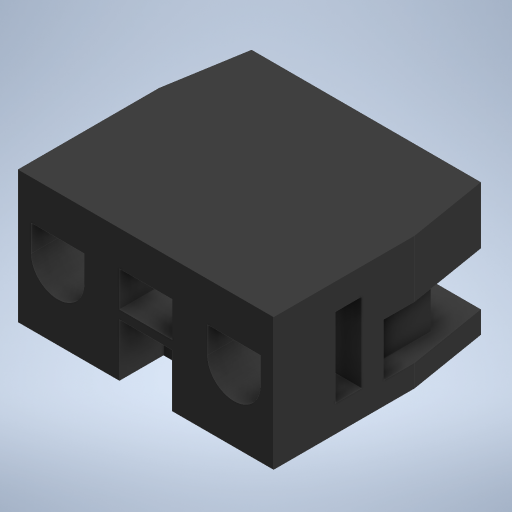
# Autodesk Inventor part: BLOCO DE CONTATO
Saved by Autodesk Inventor 2023 (Build 270158000, 158)
## iProperties
Created: 2023-10-18
Part Number: BLOCO DE CONTATO
Material: Genérico
Document SubType Name: Modeling
Designer: vinicius.sena
Density: 1 g/cm^3
Appearance: Padrão
Author: vinicius.sena
Autodesk Inventor part; units mm, degrees
ref_plane "YZ Plane" through (0, 0, 0) normal (1, 0, 0) x (0, 1, 0)
ref_plane "XZ Plane" through (0, 0, 0) normal (0, 1, 0) x (-1, 0, 0)
ref_plane "XY Plane" through (0, 0, 0) normal (0, 0, 1) x (1, 0, 0)
sketch "Esboço1" plane through (0, 0, 0) normal (0, 0, 1) x (1, 0, 0)
  line L0 (-14.5, 7.5) -> (14.5, 7.5)
  line L1 (14.5, 7.5) -> (14.5, -7.5)
  line L2 (14.5, -7.5) -> (-14.5, -7.5)
  line L3 (-14.5, -7.5) -> (-14.5, 7.5)
  line L4 (-14.5, 7.5) -> (14.5, -7.5) construction
  line L5 (14.5, 7.5) -> (-14.5, -7.5) construction
  point P0 (0, 0)
  dimension "d0" = 29
  dimension "d1" = 15
  constraints: 12 end point, 2 midpoint, 2 parallel, 1 horizontal, 1 perpendicular
  measures "d0" distance of L1.end L2.end
  measures "d1" distance of L0.end L1.end
extrude "Extrusão1" add sketch "Esboço1" along normal blind 25
sketch "Esboço2" plane through (-14.5, 7.5, 0) normal (0, 1, 0) x (1, 0, 0)
  line L0 (0, 0) -> (0, -25) projected
  line L1 (0, 0) -> (0, -9)
  line L2 (29, 0) -> (29, -25) projected
  line L3 (29, 0) -> (29, -9)
  line L4 (1.5, 0) -> (27.5, 0)
  line L5 (27.5, 0) -> (27.5, -9)
  line L6 (27.5, -9) -> (1.5, -9)
  line L7 (1.5, -9) -> (1.5, 0)
  line L8 (1.5, 0) -> (27.5, -9) construction
  line L9 (27.5, 0) -> (1.5, -9) construction
  line L10 (1.5, 0) -> (0, -9)
  line L11 (27.5, 0) -> (29, -9)
  line L12 (29, 0) -> (0, 0) projected
  line L13 (0, 0) -> (0, -25) projected
  line L14 (29, -25) -> (0, -25) projected
  line L15 (29, 0) -> (29, -25) projected
  point P0 (14.5, 0)
  point P1 (14.5, -4.5)
  dimension "d4" = 9
  dimension "d5" = 9
  dimension "d6" = 26
  constraints: 20 end point, 2 midpoint, 2 parallel, 2 point on line, 1 horizontal, 1 perpendicular
  measures "d4" distance of L0.start L1.end
  measures "d5" distance of L2.start L3.end
  measures "d6" distance of L5.end L6.end
extrude "Extrusão2" cut sketch "Esboço2" against normal through all contours L12 L10 L0 | L12 L2 L11
sketch "Esboço3" plane through (0, 0, 25) normal (0, 0, 1) x (1, 0, 0)
  circle A0 centre (10, 0) radius 3
  circle A1 centre (-10, 0) radius 3
  line L0 (-13, -7.5) -> (-13, 7.5) projected
  line L1 (-7, 3) -> (-13, 3)
  line L2 (-13, 3) -> (-13, -3)
  line L3 (-13, -3) -> (-7, -3)
  line L4 (-7, -3) -> (-7, 3)
  line L5 (-7, 3) -> (-13, -3) construction
  line L6 (-13, 3) -> (-7, -3) construction
  line L7 (13, 3) -> (7, 3)
  line L8 (7, 3) -> (7, -3)
  line L9 (7, -3) -> (13, -3)
  line L10 (13, -3) -> (13, 3)
  line L11 (13, 3) -> (7, -3) construction
  line L12 (7, 3) -> (13, -3) construction
  line L13 (3, -1.5) -> (-3, -1.5)
  line L14 (-3, -1.5) -> (-3, -7.5)
  line L15 (-3, -7.5) -> (3, -7.5)
  line L16 (3, -7.5) -> (3, -1.5)
  line L17 (3, -1.5) -> (-3, -7.5) construction
  line L18 (-3, -1.5) -> (3, -7.5) construction
  line L19 (-14.5, -7.5) -> (14.5, -7.5) projected
  point P0 (0, 0)
  point P1 (0, -4.5)
  point P2 (-7, 0)
  point P3 (-13, 0)
  point P4 (7, 0)
  point P5 (13, 0)
  dimension "d9" = 6
  dimension "d10" = 6
  dimension "d11" = 10
  dimension "d12" = 10
  dimension "d13" = 6
  dimension "d14" = 6
  dimension "d15" = 0
  constraints: 36 end point, 6 midpoint, 6 parallel, 3 horizontal, 3 perpendicular, 2 centre point, 2 point on line
  measures "d9" diameter of A0
  measures "d10" diameter of A1
  measures "d11" distance of point (0, 0) A0.centre
  measures "d12" distance of point (0, 0) A1.centre
  measures "d13" distance of L15.end L14.end
  measures "d14" distance of L14.end L13.end
  measures "d15" distance between parallel lines of L19 L15
extrude "Extrusão3" cut sketch "Esboço3" against normal blind 10 contours A0 | A0 L7 L10 | A0 L8 L7 | A1 | A1 L1 L4 | A1 L0 L1
sketch "Esboço4" plane through (-14.5, -7.5, 25) normal (-1, 0, 0) x (0, 0, 1)
  line L0 (-7, 12) -> (-10, 12)
  line L1 (-10, 12) -> (-10, 3)
  line L2 (-10, 3) -> (-7, 3)
  line L3 (-7, 3) -> (-7, 12)
  line L4 (-7, 12) -> (-10, 3) construction
  line L5 (-10, 12) -> (-7, 3) construction
  line L6 (-10, 7.5) -> (-10, 10.5) projected
  point P0 (-25, 7.5)
  point P1 (-8.5, 7.5)
  dimension "d18" = 3
  dimension "d19" = 9
  dimension "d20" = 0
  constraints: 12 end point, 3 midpoint, 2 parallel, 1 horizontal, 1 perpendicular
  measures "d18" distance of L2.end L1.end
  measures "d19" distance of L1.end L0.end
  measures "d20" distance from line of L6 point (-10, 7.5)
extrude "Extrusão4" cut sketch "Esboço4" against normal blind 7.5
sketch "Esboço5" plane through (14.5, -7.5, 25) normal (1, 0, 0) x (0, 0, -1)
  line L0 (7, 3) -> (10, 3)
  line L1 (10, 3) -> (10, 12)
  line L2 (10, 12) -> (7, 12)
  line L3 (7, 12) -> (7, 3)
  line L4 (0, 7.5) -> (10, 7.5) projected
  line L5 (7, 3) -> (10, 12) construction
  line L6 (10, 3) -> (7, 12) construction
  line L7 (10, 4.5) -> (10, 7.5) projected
  point P0 (25, 7.5)
  point P1 (8.5, 7.5)
  dimension "d23" = 3
  dimension "d24" = 9
  dimension "d25" = 0
  constraints: 12 end point, 2 midpoint, 2 parallel, 1 horizontal, 1 perpendicular, 1 point on line
  measures "d23" distance of L2.end L1.end
  measures "d24" distance of L1.end L0.end
  measures "d25" distance between parallel lines of L7 L1
extrude "Extrusão5" cut sketch "Esboço5" against normal blind 7.5
sketch "Esboço6" plane through (0, 0, 25) normal (0, 0, 1) x (1, 0, 0)
  line L0 (-3, -7.5) -> (3, -7.5)
  line L1 (3, -7.5) -> (3, -1.5)
  line L2 (3, -1.5) -> (-3, -1.5)
  line L3 (-3, -1.5) -> (-3, -7.5)
  line L4 (-3, -7.5) -> (3, -1.5) construction
  line L5 (3, -7.5) -> (-3, -1.5) construction
  line L6 (-14.5, -7.5) -> (14.5, -7.5) projected
  line L7 (-3, -0.5) -> (3, -0.5)
  line L8 (3, -0.5) -> (3, 3.5)
  line L9 (3, 3.5) -> (-3, 3.5)
  line L10 (-3, 3.5) -> (-3, -0.5)
  line L11 (-3, -0.5) -> (3, 3.5) construction
  line L12 (3, -0.5) -> (-3, 3.5) construction
  point P0 (0, 0)
  point P1 (0, -4.5)
  point P2 (0, 1.5)
  dimension "d28" = 6
  dimension "d29" = 6
  dimension "d30" = 0
  dimension "d31" = 6
  dimension "d32" = 4
  constraints: 24 end point, 4 midpoint, 4 parallel, 2 horizontal, 2 perpendicular
  measures "d28" distance of L2.end L1.end
  measures "d29" distance of L1.end L0.end
  measures "d30" distance between parallel lines of L6 L0
  measures "d31" distance of L9.end L8.end
  measures "d32" distance of L8.end L7.end
extrude "Extrusão6" cut sketch "Esboço6" against normal blind 5
sketch "Esboço8" plane through (0, 0, 20) normal (0, 0, 1) x (1, 0, 0)
  line L0 (3, -7.5) -> (-3, -7.5) projected
  point P0 (0, 0)
  point P1 (0, -5.5)
  point P2 (0, -7.5)
  dimension "d42" = 2
  dimension "d43" = 0
  constraints: 1 midpoint
  measures "d42" distance of point (0, -7.5) point (0, -5.5)
  measures "d43" horizontal distance of point (0, 0) point (0, -5.5)
hole "Furo1" at (0, -5.5, 20) direction (0, 0, -1) diameter 3 end through all
sketch "Esboço9" plane through (0, 0, 0) normal (0, 0, -1) x (-1, 0, 0)
  circle A0 centre (0, -5.5) radius 1.5 projected
  circle A1 centre (0, -5.5) radius 2.5
  line L0 (2.5, -5.5) -> (2.5, -7.5)
  line L1 (13, -7.5) -> (-13, -7.5) projected
  line L2 (-2.5, -5.5) -> (-2.5, -7.5)
  line L3 (2.5, -7.5) -> (-2.5, -7.5)
  point P0 (0, 0)
  point P1 (-1.5, -7.5)
  point P2 (1.5, -7.5)
  point P3 (-1.5, -7.5)
  dimension "d44" = 5
  constraints: 6 end point, 2 point on circle, 2 point on line, 1 centre point, 1 coincident, 1 parallel, 1 perpendicular, 1 vertical
  measures "d44" diameter of A1
extrude "Extrusão7" cut sketch "Esboço9" against normal blind 1 contours A1 L1 | L0 L1 A1 | A1 L1 L2 picked at (0.0603, -7.3297)
sketch "Esboço10" plane through (0, 0, 0) normal (0, 0, -1) x (-1, 0, 0)
  line L0 (14.5, 1) -> (7.5, 1)
  line L1 (7.5, 1) -> (7.5, -5)
  line L2 (7.5, -5) -> (14.5, -5)
  line L3 (14.5, -5) -> (14.5, 1)
  line L4 (14.5, 1) -> (7.5, -5) construction
  line L5 (7.5, 1) -> (14.5, -5) construction
  line L6 (14.5, 7.5) -> (14.5, -7.5) projected
  line L7 (13, -7.5) -> (2.5, -7.5) projected
  line L8 (-7.5, 1) -> (-14.5, 1)
  line L9 (-14.5, 1) -> (-14.5, -5)
  line L10 (-14.5, -5) -> (-7.5, -5)
  line L11 (-7.5, -5) -> (-7.5, 1)
  line L12 (-7.5, 1) -> (-14.5, -5) construction
  line L13 (-14.5, 1) -> (-7.5, -5) construction
  line L14 (-14.5, -7.5) -> (-14.5, 7.5) projected
  line L15 (-2.5, -7.5) -> (-13, -7.5) projected
  point P0 (0, 0)
  point P1 (11, -2)
  point P2 (11, -5)
  point P3 (-11, -2)
  dimension "d47" = 7
  dimension "d48" = 6
  dimension "d49" = 0
  dimension "d50" = 2.5
  dimension "d51" = 7
  dimension "d52" = 6
  dimension "d53" = 0
  dimension "d54" = 2.5
  constraints: 24 end point, 5 midpoint, 4 parallel, 2 horizontal, 2 perpendicular
  measures "d47" distance of L2.end L1.end
  measures "d48" distance of L1.end L0.end
  measures "d49" distance between parallel lines of L6 L3
  measures "d50" distance from line of L7 point (11, -5)
  measures "d51" distance of L10.end L9.end
  measures "d52" distance of L9.end L8.end
  measures "d53" distance between parallel lines of L14 L9
  measures "d54" distance between parallel lines of L15 L10
extrude "Extrusão8" cut sketch "Esboço10" against normal blind 5
sketch "Esboço11" plane through (0, 0, 5) normal (0, 0, -1) x (-1, 0, 0)
  line L0 (15.3333, 1) -> (12.3333, 1)
  line L1 (12.3333, 1) -> (12.3333, -5)
  line L2 (12.3333, -5) -> (15.3333, -5)
  line L3 (15.3333, -5) -> (15.3333, 1)
  line L4 (13.8333, 1) -> (13.8333, -5) projected
  line L5 (15.3333, 1) -> (12.3333, -5) construction
  line L6 (12.3333, 1) -> (15.3333, -5) construction
  line L7 (-12.3333, 1) -> (-15.3333, 1)
  line L8 (-15.3333, 1) -> (-15.3333, -5)
  line L9 (-15.3333, -5) -> (-12.3333, -5)
  line L10 (-12.3333, -5) -> (-12.3333, 1)
  line L11 (-13.8333, -5) -> (-13.8333, 1) projected
  line L12 (-12.3333, 1) -> (-15.3333, -5) construction
  line L13 (-15.3333, 1) -> (-12.3333, -5) construction
  point P0 (0, 0)
  point P1 (13.8333, -2)
  point P2 (-13.8333, -2)
  dimension "d57" = 3
  dimension "d58" = 6
  dimension "d59" = 3
  dimension "d60" = 6
  constraints: 24 end point, 6 midpoint, 4 parallel, 2 horizontal, 2 perpendicular
  measures "d57" distance of L2.end L1.end
  measures "d58" distance of L1.end L0.end
  measures "d59" distance of L9.end L8.end
  measures "d60" distance of L8.end L7.end
extrude "Extrusão9" cut sketch "Esboço11" against normal blind 7.5
sketch "Esboço12" plane through (0, 0, 15) normal (0, 0, 1) x (1, 0, 0)
  arc A0 (7, 0) -> (13, 0) centre (10, 0) ccw projected
  arc A1 (-13, 0) -> (-7, 0) centre (-10, 0) ccw projected
  point P0 (0, 0)
  dimension "d70" = 0
  dimension "d71" = 0
  dimension "d72" = 0
  dimension "d73" = 0
  measures "d70" distance of A0.centre point (10, 0)
  measures "d71" distance of A0.centre point (10, 0)
  measures "d72" distance of A1.centre point (-10, 0)
  measures "d73" distance of A1.centre point (-10, 0)
hole "Furo2" at (10, 0, 15) at (-10, 0, 15) direction (0, 0, -1) diameter 3 depth 0.998 tip angle 118
sketch "Esboço14" plane through (0, 0, 20) normal (0, 0, 1) x (1, 0, 0)
  line L0 (3, 3.5) -> (3, -0.5) projected
  line L1 (-3, 3.5) -> (3, 3.5) projected
  line L2 (-3, -0.5) -> (-3, 3.5) projected
  line L3 (3, -0.5) -> (-3, -0.5) projected
  point P0 (0, 0)
extrude "Extrusão11" cut sketch "Esboço14" against normal through all
